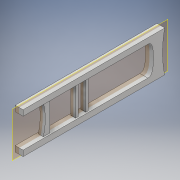
# Autodesk Inventor part: main_tower
Saved by Autodesk Inventor 2017 (Build 210142000, 142)
## iProperties
Part Number: main_tower
Material: 一般
Document SubType Name: Modeling
Designer: 3890237626
Density: 1 g/cm^3
Appearance: 既定
Author: 3890237626
Autodesk Inventor part; units mm, degrees
ref_plane "YZ Plane" through (0, 0, 0) normal (1, 0, 0) x (0, 1, 0)
ref_plane "XZ Plane" through (0, 0, 0) normal (0, 1, 0) x (-1, 0, 0)
ref_plane "XY Plane" through (0, 0, 0) normal (0, 0, 1) x (1, 0, 0)
sketch "スケッチ1" plane through (0, 0, 0) normal (1, 0, 0) x (0, 1, 0)
  line L0 (14648.4771, -87001.3054) -> (-110951.5229, -87001.3054)
  line L1 (-110951.5229, -87001.3054) -> (-110951.5229, -92001.3054)
  line L2 (-110951.5229, -92001.3054) -> (-351.5229, -92001.3054)
  spline S0 degree 4 poles (-351.5229, -92001.3054) (3276.1521, -92001.3054) (4991.3905, -99504.2453) (4991.3905, -110498.3655) (3276.1521, -118001.3054) (-351.5229, -118001.3054) knots 0 0 0 0 0 0.5 1 1 1 1 1
  line L3 (-351.5229, -118001.3054) -> (-110951.5229, -118001.3054)
  line L4 (-110951.5229, -118001.3054) -> (-110951.5229, -123001.3054)
  line L5 (-110951.5229, -123001.3054) -> (14648.4771, -123001.3054)
  spline S1 degree 3 poles (14648.4771, -87001.3054) (12017.7135, -95778.8229) (12017.7135, -114223.7879) (14648.4771, -123001.3054) knots 0 0 0 0 1 1 1 1
  point P0 (0, 0)
  point P1 (4033.3753, -97539.5737)
  point P2 (4033.3753, -112463.0371)
  point P3 (12947.7718, -97539.5737)
  point P4 (12947.7718, -112463.0371)
  dimension "d0" = 125600
  dimension "d1" = 5000
  dimension "d2" = 36000
  dimension "d3" = 15000
  dimension "d4" = 4384.8982
  dimension "d5" = 1700.7053
  dimension "d6" = 5538.2683
  dimension "d7" = 5538.2683
  constraints: 12 end point, 4 horizontal, 4 perpendicular, 4 vertical alignment, 2 collinear, 2 horizontal alignment, 8 other
  measures "d0" distance of L4.end L5.end
  measures "d1" distance of L3.end L4.end
  measures "d2" distance of L0.start L5.end
  measures "d3" horizontal distance of L3.start L5.end
  measures "d4" horizontal distance of L3.start point (4033.375, -112463.037)
  measures "d5" horizontal distance of L5.end point (12947.772, -112463.037)
  measures "d6" vertical distance of L2.end point (4033.375, -97539.574)
  measures "d7" vertical distance of L3.start point (4033.375, -112463.037)
extrude "押し出し1" add sketch "スケッチ1" along normal blind 7000
ref_plane "作業平面1" through (3500, 0, 0) normal (1, 0, 0) x (0, 0, -1)
sketch "スケッチ2" plane through (3500, 0, 0) normal (1, 0, 0) x (0, 0, -1)
  line L0 (87001.3054, 14648.4771) -> (87001.3054, -110951.5229) projected
  line L1 (87001.3054, -110951.5229) -> (92001.3054, -110951.5229) projected
  line L2 (92001.3054, -110951.5229) -> (92001.3054, -351.5229) projected
  line L3 (118001.3054, -351.5229) -> (118001.3054, -110951.5229) projected
  line L4 (118001.3054, -110951.5229) -> (123001.3054, -110951.5229) projected
  line L5 (123001.3054, -110951.5229) -> (123001.3054, 14648.4771) projected
  line L6 (87001.3054, 14648.4771) -> (87001.3054, -110951.5229) projected
  arc A0 (118001.3054, -91751.5229) -> (92001.3054, -91751.5229) centre (105001.3054, -140268.1834) ccw
  line L7 (92001.3054, -110951.5229) -> (92001.3054, -351.5229) projected
  line L8 (118001.3054, -351.5229) -> (118001.3054, -110951.5229) projected
  line L9 (117801.3054, -85951.5229) -> (92201.3054, -85951.5229)
  line L10 (92201.3054, -85951.5229) -> (92001.3054, -85751.5229)
  line L11 (117801.3054, -85951.5229) -> (118001.3054, -85751.5229)
  line L12 (92001.3054, -91751.5229) -> (92001.3054, -85751.5229)
  line L13 (118001.3054, -91751.5229) -> (118001.3054, -85751.5229)
  line L14 (92201.3054, -62951.5229) -> (117801.3054, -62951.5229)
  line L15 (117801.3054, -62951.5229) -> (118001.3054, -63151.5229)
  line L16 (92201.3054, -62951.5229) -> (92001.3054, -63151.5229)
  line L17 (118001.3054, -63151.5229) -> (118001.3054, -60951.5229)
  line L18 (118001.3054, -60951.5229) -> (92001.3054, -60951.5229)
  line L19 (92001.3054, -60951.5229) -> (92001.3054, -63151.5229)
  line L20 (92001.3054, -51951.5229) -> (92001.3054, -54151.5229)
  line L21 (118001.3054, -51951.5229) -> (92001.3054, -51951.5229)
  line L22 (92201.3054, -53951.5229) -> (92001.3054, -54151.5229)
  line L23 (92201.3054, -53951.5229) -> (117801.3054, -53951.5229)
  line L24 (118001.3054, -54151.5229) -> (118001.3054, -51951.5229)
  line L25 (117801.3054, -53951.5229) -> (118001.3054, -54151.5229)
  point P0 (0, 0)
  dimension "d11" = 30
  dimension "d12" = 200
  dimension "d13" = 200
  dimension "d14" = 6000
  dimension "d15" = 25000
  dimension "d16" = 200
  dimension "d17" = 200
  dimension "d18" = 2000
  dimension "d19" = 50000
  dimension "d20" = 200
  dimension "d23" = 9000
  constraints: 34 end point, 5 horizontal alignment, 4 point on line, 3 collinear, 3 vertical, 2 horizontal, 2 perpendicular, 2 point on circle, 1 centre point, 12 other
  measures "d12" distance from line of L2 L9.end
  measures "d13" horizontal distance of L9.end L10.end
  measures "d14" distance of L12.start L10.end
  measures "d15" distance between parallel lines of L4 L9
  measures "d16" horizontal distance of L16.end L14.start
  measures "d17" horizontal distance of L16.end L14.start
  measures "d18" distance between parallel lines of L14 L18
  measures "d19" distance between parallel lines of L4 L18
  measures "d20" horizontal distance of L15.end L14.end
  measures "d23" distance of L18.end L20.start
extrude "押し出し2" add sketch "スケッチ2" along normal mid plane 4500 contours L2 L10 L9 L11 L3 A0 | L2 L18 L3 L15 L14 L16 | L2 L21 L3 L25 L23 L22
equation "\"d7\" = d6"
equation "\"d12\" = d13"
equation "\"d16\" = d17"
equation "\"d17\" = d13"
equation "\"d20\" = d17"
